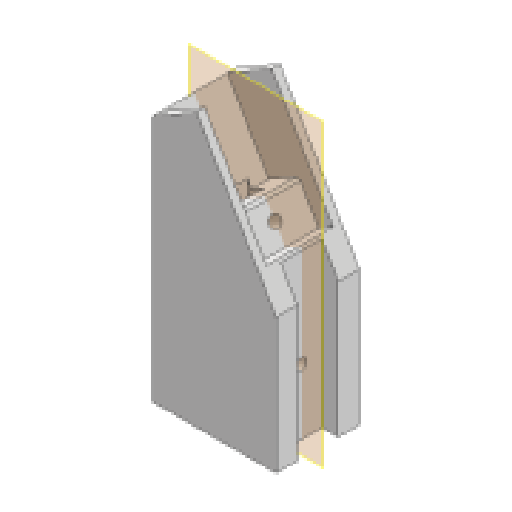
# Autodesk Inventor part: PALM 2
Saved by Autodesk Inventor 2025.1 (Build 291241020, 241B)
## iProperties
Created: 2024-12-04
Part Number: PALM 2
Material: Generic
Document SubType Name: Modeling
Designer: ALEXANDERNICHOLS
Density: 1 g/cm^3
Appearance: Default
Author: ALEXANDERNICHOLS
Autodesk Inventor part; units mm, degrees
ref_plane "YZ Plane" through (0, 0, 0) normal (1, 0, 0) x (0, 1, 0)
ref_plane "XZ Plane" through (0, 0, 0) normal (0, 1, 0) x (-1, 0, 0)
sketch "Sketch1" plane through (0, 0, 0) normal (0, 0, 1) x (1, 0, 0)
  line L0 (0, 0) -> (38.1, 0)
  line L1 (38.1, 0) -> (38.1, 41.6033)
  line L2 (0, 76.2) -> (0, 0)
  line L3 (0, 76.2) -> (13.5942, 84.0486)
  line L4 (0, 76.2) -> (12.7, 54.203)
  line L5 (12.7, 54.203) -> (26.2942, 62.0516)
  line L6 (26.2942, 62.0516) -> (13.5942, 84.0486)
  line L7 (26.2942, 62.0516) -> (38.1, 41.6033)
  dimension "d0" = 15.6972
  dimension "d1" = 25.4
  dimension "d2" = 38.1
  dimension "d3" = 76.2
  dimension "d4" = 120
  constraints: 16 end point, 4 perpendicular, 2 point on line, 1 collinear, 1 horizontal, 1 parallel
  measures "d0" distance between parallel lines of L4 L6
  measures "d1" distance between parallel lines of L5 L3
  measures "d2" distance of L0.start L0.end
  measures "d3" distance from line of L2.start L0
  measures "d4" angle of L2 L3
extrude "Extrusion1" add sketch "Sketch1" along normal blind 20.574 contours L2 L4 L5 L7 L1 L0
sketch "Sketch2" plane through (0, 0, 20.574) normal (0, 0, 1) x (1, 0, 0)
  line L0 (0, 76.2) -> (0, 0) projected
  line L1 (0, 0) -> (38.1, 0) projected
  line L2 (38.1, 0) -> (38.1, 41.6033) projected
  line L3 (38.1, 41.6033) -> (26.2942, 62.0516) projected
  line L4 (26.2942, 62.0516) -> (12.7, 54.203) projected
  line L5 (12.7, 54.203) -> (0, 76.2) projected
  line L6 (26.2942, 62.0516) -> (13.5942, 84.0486)
  line L7 (13.5942, 84.0486) -> (0, 76.2)
  line L8 (38.1, 41.6033) -> (26.2942, 62.0516) projected
  constraints: 4 end point, 1 collinear, 1 perpendicular
extrude "Extrusion2" add sketch "Sketch2" along normal blind 2.54
ref_plane "Work Plane1" through (0, 0, 10.287) normal (0, 0, -1) x (-1, 0, 0)
mirror "Mirror1" about plane through (0, 0, 10.287) normal (0, 0, -1) of "Extrusion2"
sketch "Sketch3" plane through (0, 0, 23.114) normal (0, -1, 0) x (1, 0, 0)
  line L0 (38.1, -25.654) -> (38.1, 0) projected
  line L1 (38.1, -6.477) -> (33.02, -6.477)
  line L2 (33.02, -6.477) -> (33.02, -19.177)
  line L3 (33.02, -19.177) -> (38.1, -19.177)
  line L4 (38.1, -19.177) -> (38.1, -6.477)
  point P0 (0, -23.114)
  point P1 (38.1, -12.827)
  point P2 (38.1, -19.177)
  dimension "d9" = 12.7
  dimension "d10" = 6.35
  dimension "d11" = 5.08
  constraints: 8 end point, 2 parallel, 1 horizontal, 1 midpoint, 1 perpendicular, 1 point on line
  measures "d9" distance between parallel lines of L3 L1
  measures "d10" distance from line of point (38.1, -12.827) L3
  measures "d11" distance between parallel lines of L0 L2
extrude "Extrusion3" cut sketch "Sketch3" against normal blind 65.0875
sketch "Sketch4" plane through (33.02, 0, 16.637) normal (1, 0, 0) x (0, 0, -1)
  circle A0 centre (6.35, 20.122) radius 1.778 projected
  point P0 (16.637, 0)
extrude "Extrusion4" cut sketch "Sketch4" against normal blind 15.24
sketch "Sketch5" plane through (13.5942, 84.0486, 23.114) normal (0.8660254, 0.5, 0) x (0, 0, -1)
  line L0 (23.114, -25.4) -> (2.54, -25.4) projected
  line L1 (23.114, -25.4) -> (2.54, -25.4)
  line L2 (2.54, -25.4) -> (2.54, -37.7698)
  line L3 (2.54, -37.7698) -> (23.114, -37.7698)
  line L4 (23.114, -37.7698) -> (23.114, -25.4)
  point P0 (23.114, -65.9911)
  dimension "d16" = 12.3698
  constraints: 8 end point, 2 parallel, 1 horizontal, 1 perpendicular
  measures "d16" distance between parallel lines of L3 L0
extrude "Extrusion5" cut sketch "Sketch5" against normal blind 5.08
chamfer "Chamfer1" distance 1.016 angle 45 1 edges at (21.893, 59.5106, 10.287)
sketch "Sketch6" plane through (9.1948, 81.5086, 23.114) normal (0.8660254, 0.5, 0) x (0, 0, -1)
  line L0 (2.54, -39.2429) -> (2.54, -0.5012) projected
  line L1 (2.54, -25.4) -> (22.86, -25.4) projected
  line L2 (23.114, -37.7698) -> (2.54, -37.7698) projected
  line L3 (2.54, -37.7698) -> (2.54, 0) projected
  line L4 (2.54, -25.4) -> (2.54, -37.7698)
  circle A0 centre (12.827, -31.5849) radius 1.778
  line L5 (23.114, -37.7698) -> (2.54, -37.7698) projected
  point P0 (23.114, -65.9911)
  point P1 (2.54, -31.5849)
  point P2 (12.827, -37.7698)
  dimension "d22" = 3.556
  constraints: 2 end point, 2 midpoint, 1 centre point, 1 collinear, 1 horizontal alignment, 1 vertical alignment
  measures "d22" diameter of A0
extrude "Extrusion6" cut sketch "Sketch6" against normal blind 7.62
ref_plane "Work Plane2" through (0, 0, 10.287) normal (0, 0, 1) x (1, 0, 0)
sketch "Sketch7" plane through (0, 0, 10.287) normal (0, 0, 1) x (1, 0, 0)
  line L0 (21.0149, 59.0036) -> (12.7, 54.203) projected
  line L1 (16.51, 56.4027) -> (11.43, 56.4027)
  line L2 (12.7, 54.203) -> (0, 76.2) projected
  line L3 (16.51, 56.4027) -> (16.51, 0)
  line L4 (0, 0) -> (38.1, 0) projected
  line L5 (11.43, 56.4027) -> (11.43, 0)
  line L6 (11.43, 0) -> (16.51, 0)
  dimension "d25" = 5.08
  constraints: 8 end point, 4 point on line, 1 collinear, 1 horizontal, 1 parallel, 1 vertical
  measures "d25" distance between parallel lines of L5 L3
extrude "Extrusion7" cut sketch "Sketch7" along normal mid plane 10.16 contours L3 L4 L5 L2 L0
sketch "Sketch8" plane through (0, 0, 23.114) normal (-1, 0, 0) x (0, 0, 1)
  circle A0 centre (-12.827, 44.45) radius 1.778 projected
  circle A1 centre (-12.827, 19.05) radius 1.778 projected
  point P0 (-23.114, 0)
extrude "Extrusion8" cut sketch "Sketch8" against normal blind 15.24
sketch "Sketch9" plane through (0, 0, 23.114) normal (0, -1, 0) x (1, 0, 0)
  circle A0 centre (5.08, -12.827) radius 1.778 projected
  circle A1 centre (22.86, -12.827) radius 1.778 projected
  point P0 (0, -23.114)
extrude "Extrusion9" cut sketch "Sketch9" against normal blind 15.24
equation "\"d10\" = 0.5 * d9"
body "Solid1"
